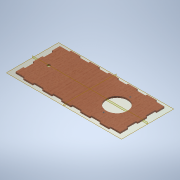
# Autodesk Inventor part: Plaat boven
Saved by Autodesk Inventor 2021 (Build 250183000, 183)
## iProperties
Manager: PJ / DCS
Company: Emmaüs Bovenbouw Aalter
Created: 2021-01-09
Part Number: Plaat boven
Material: S235
Catalog Web Link: http://emmausbovenbouw.op-weg.be/
Vendor: Emmaüsinstituut Bovenbouw Aalter
Document SubType Name: Modeling
Designer: Antho
Engineer: Declercq St.
Manufacturer: Standard
Standards Organization: Custom
Density: 7.86 g/cm^3
Appearance: Steel
Title: Algemene titel
Subject: Specifieke titel
Author: Antho
Keywords: Ruwe Ø xxxxx
Comments: Opmerking
Autodesk Inventor part; units mm, degrees
sketch "Sketch1" plane through (0, 0, 0) normal (0, 0, 1) x (1, 0, 0)
  line L0 (0, 2.8582) -> (0, -2.8582) construction
  line L1 (-5.7775, 0) -> (5.7775, 0) construction
  line L2 (-165, -75) -> (165, -75)
  line L3 (165, -75) -> (165, 75)
  line L4 (165, 75) -> (-165, 75)
  line L5 (-165, 75) -> (-165, -75)
  line L6 (-165, -75) -> (165, 75) construction
  line L7 (165, -75) -> (-165, 75) construction
  point P0 (0, 0)
  point P1 (0, 0)
  dimension "d0" = 330
  dimension "d1" = 150
  constraints: 16 end point, 4 midpoint, 2 horizontal, 2 parallel, 1 coincident, 1 perpendicular, 1 vertical
  measures "d0" distance of L4.end L3.end
  measures "d1" distance of L3.end L2.end
extrude "Extrusion1" add sketch "Sketch1" along normal blind 5
sketch "Sketch2" plane through (0, 0, 5) normal (0, 0, 1) x (1, 0, 0)
  line L0 (0, 0) -> (-130, 0)
  circle A0 centre (-130, 0) radius 5
  line L1 (-165, 75) -> (-165, -75) projected
  line L2 (-165, 0) -> (-165, 15)
  line L3 (-165, 15) -> (-165, -15)
  line L4 (-165, -15) -> (-165, -45)
  line L5 (-165, -45) -> (-165, -75)
  line L6 (-165, 15) -> (-165, 45)
  line L7 (-165, 45) -> (-165, 75)
  line L8 (-165, 15) -> (-160, 15)
  line L9 (-160, 15) -> (-160, 45)
  line L10 (-160, 45) -> (-165, 45)
  line L11 (-165, 45) -> (-165, 15)
  line L12 (-165, -15) -> (-160, -15)
  line L13 (-160, -15) -> (-160, -45)
  line L14 (-160, -45) -> (-165, -45)
  line L15 (-165, -45) -> (-165, -15)
  line L16 (-165, -75) -> (165, -75) projected
  line L17 (-165, -75) -> (-135, -75)
  line L18 (-135, -75) -> (-105, -75)
  line L19 (-105, -75) -> (-75, -75)
  line L20 (-75, -75) -> (-45, -75)
  line L21 (-45, -75) -> (-15, -75)
  line L22 (-15, -75) -> (15, -75)
  line L23 (15, -75) -> (45, -75)
  line L24 (45, -75) -> (75, -75)
  line L25 (75, -75) -> (105, -75)
  line L26 (105, -75) -> (135, -75)
  line L27 (135, -75) -> (165, -75)
  line L28 (-165, -75) -> (-135, -75)
  line L29 (-135, -75) -> (-135, -70)
  line L30 (-135, -70) -> (-165, -70)
  line L31 (-165, -70) -> (-165, -75)
  line L32 (-105, -75) -> (-75, -75)
  line L33 (-75, -75) -> (-75, -70)
  line L34 (-75, -70) -> (-105, -70)
  line L35 (-105, -70) -> (-105, -75)
  line L36 (-45, -75) -> (-15, -75)
  line L37 (-15, -75) -> (-15, -70)
  line L38 (-15, -70) -> (-45, -70)
  line L39 (-45, -70) -> (-45, -75)
  line L40 (15, -75) -> (45, -75)
  line L41 (45, -75) -> (45, -70)
  line L42 (45, -70) -> (15, -70)
  line L43 (15, -70) -> (15, -75)
  line L44 (75, -75) -> (105, -75)
  line L45 (105, -75) -> (105, -70)
  line L46 (105, -70) -> (75, -70)
  line L47 (75, -70) -> (75, -75)
  line L48 (135, -75) -> (165, -75)
  line L49 (165, -75) -> (165, -70)
  line L50 (165, -70) -> (135, -70)
  line L51 (135, -70) -> (135, -75)
  line L52 (165, 75) -> (-165, 75) projected
  line L53 (-165, 75) -> (-135, 75)
  line L54 (-135, 75) -> (-135, 70)
  line L55 (-135, 70) -> (-165, 70)
  line L56 (-165, 70) -> (-165, 75)
  line L57 (-105, 75) -> (-75, 75)
  line L58 (-75, 75) -> (-75, 70)
  line L59 (-75, 70) -> (-105, 70)
  line L60 (-105, 70) -> (-105, 75)
  line L61 (-45, 75) -> (-15, 75)
  line L62 (-15, 75) -> (-15, 70)
  line L63 (-15, 70) -> (-45, 70)
  line L64 (-45, 70) -> (-45, 75)
  line L65 (15, 75) -> (45, 75)
  line L66 (45, 75) -> (45, 70)
  line L67 (45, 70) -> (15, 70)
  line L68 (15, 70) -> (15, 75)
  line L69 (75, 75) -> (105, 75)
  line L70 (105, 75) -> (105, 70)
  line L71 (105, 70) -> (75, 70)
  line L72 (75, 70) -> (75, 75)
  line L73 (165, -75) -> (165, 75) projected
  line L74 (135, 75) -> (165, 75)
  line L75 (165, 75) -> (165, 70)
  line L76 (165, 70) -> (135, 70)
  line L77 (135, 70) -> (135, 75)
  line L78 (165, 0) -> (165, 15)
  line L79 (165, 15) -> (160, 15)
  line L80 (160, 15) -> (160, 45)
  line L81 (160, 45) -> (165, 45)
  line L82 (165, 45) -> (165, 15)
  line L83 (165, -15) -> (160, -15)
  line L84 (160, -15) -> (160, -45)
  line L85 (160, -45) -> (165, -45)
  line L86 (165, -45) -> (165, -15)
  point P0 (-165, -70)
  point P1 (135, 75)
  point P2 (105, 75)
  point P3 (75, 75)
  point P4 (45, 75)
  point P5 (15, 75)
  point P6 (-15, 75)
  point P7 (-165, 70)
  point P8 (-165, -45)
  dimension "d4" = 130
  dimension "d5" = 10
  dimension "d6" = 15
  dimension "d7" = 30
  dimension "d8" = 30
  dimension "d9" = 30
  dimension "d10" = 30
  dimension "d11" = 30
  dimension "d12" = 5
  dimension "d13" = 30
  dimension "d14" = 30
  dimension "d15" = 30
  dimension "d16" = 30
  dimension "d17" = 30
  dimension "d18" = 30
  dimension "d19" = 30
  dimension "d20" = 30
  dimension "d21" = 30
  dimension "d22" = 30
  dimension "d23" = 30
  dimension "d24" = 5
  dimension "d25" = 5
  dimension "d26" = 5
  dimension "d29" = 30
  dimension "d30" = 30
  dimension "d31" = 30
  dimension "d32" = 30
  dimension "d33" = 30
  dimension "d34" = 30
  constraints: 166 end point, 35 point on line, 32 parallel, 17 horizontal, 16 perpendicular, 2 collinear, 2 midpoint, 1 centre point, 1 coincident, 11 other
  measures "d4" distance of L0.start L0.end
  measures "d5" diameter of A0
  measures "d6" distance of L2.start L2.end
  measures "d7" distance of L2.end L3.end
  measures "d8" distance of L3.end L4.end
  measures "d9" distance of L4.end L1.end
  measures "d10" distance of L2.end L6.end
  measures "d11" distance of L6.end L1.start
  measures "d12" distance of L10.end L9.end
  measures "d13" distance of L1.end L17.end
  measures "d14" distance of L17.end L18.end
  measures "d15" distance of L18.end L19.end
  measures "d16" distance of L19.end L20.end
  measures "d17" distance of L20.end L21.end
  measures "d18" distance of L21.end L22.end
  measures "d19" distance of L22.end L23.end
  measures "d20" distance of L23.end L24.end
  measures "d21" distance of L24.end L25.end
  measures "d22" distance of L25.end L26.end
  measures "d23" distance of L26.end L27.end
  measures "d24" distance of L29.end L28.end
  measures "d25" distance of L53.end L54.end
  measures "d26" distance of L80.end L81.end
  measures "d29" distance of L29.end L30.end
  measures "d30" distance of L33.end L34.end
  measures "d31" distance of L37.end L38.end
  measures "d32" distance of L41.end L42.end
  measures "d33" distance of L45.end L46.end
  measures "d34" distance of L49.end L50.end
extrude "Extrusion2" cut sketch "Sketch2" against normal blind 5 contours A0 | L52 L54 L55 L1 | L10 L9 L8 L1 | L52 L58 L59 L60 | L52 L62 L63 L64 | L12 L13 L14 L1 | L52 L66 L67 L68 | L30 L29 L16 L1 | L52 L70 L71 L72 | L35 L34 L33 L16 | L52 L73 L76 L77 | L39 L38 L37 L16 | L73 L79 L80 L81 | L43 L42 L41 L16 | L47 L46 L45 L16 | L73 L85 L84 L83 | L51 L50 L49 L16
sketch "Sketch3" plane through (0, 0, 5) normal (0, 0, 1) x (1, 0, 0)
  line L0 (165, -15) -> (165, 15) projected
  line L1 (165, 0) -> (85, 0)
  circle A0 centre (85, 0) radius 33.5
  point P0 (0, 0)
  dimension "d35" = 80
  dimension "d36" = 67
  constraints: 2 end point, 1 centre point, 1 coincident, 1 horizontal, 1 midpoint
  measures "d35" distance of L1.start L1.end
  measures "d36" diameter of A0
extrude "Extrusion3" cut sketch "Sketch3" against normal blind 10
sketch "Sketch4" plane through (0, 0, 5) normal (0, 0, 1) x (1, 0, 0)
  circle A0 centre (85, 0) radius 33.5 projected
  line L0 (85, 0) -> (85, 42)
  circle A1 centre (85, 42) radius 2.5
  line L1 (85, 0) -> (85, -42)
  circle A2 centre (85, -42) radius 2.5
  point P0 (0, 0)
  dimension "d39" = 42
  dimension "d40" = 5
  dimension "d41" = 42
  dimension "d42" = 5
  constraints: 4 end point, 2 centre point, 2 coincident, 2 vertical
  measures "d39" distance of L0.start L0.end
  measures "d40" diameter of A1
  measures "d41" distance of L0.start L1.end
  measures "d42" diameter of A2
extrude "Extrusion4" cut sketch "Sketch4" against normal blind 5 contours A1 | A2
body "Solid1"
